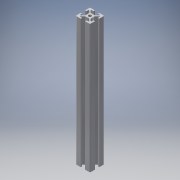
# Autodesk Inventor part: NFS5-2020-200
Saved by Autodesk Inventor 2016 (Build 200138000, 138)
## iProperties
Category: PARTsolutions
Company: MISUMI
Created: 2016-06-28
Part Number: NFS5-2020-200
Catalog Web Link: www.cadenas.de
Description: NFS5-2020, NFSB5-2020, HFS5-2020, HFSB5-2020, CAF5-2020, HFSY5-2020, NFSF5-2020, HFSF5-2020, HFSFB5-2020, NFST5-2020, HFST5-2020, HFSTB5-2020, HFSH5-2020, HFSC5-2020-HFS5 Series Aluminum Extrusions 20 Square -1 Slot-
Vendor: MISUMI
Document SubType Name: Modeling
Designer: psAdmin
Manufacturer: MISUMI
Mass: 36.2526 g
Surface Area: 351.759 cm^2
Volume: 36.2526 cm^3
Density: 2.7 g/cm^3
Material: アルミニウム 6061
Appearance: アルミニウム - フラット
PSOL_IDENT_0: {$CADENAS_DATA\23d-libs\misumi\metric\38_al_extrusions_blackets\5\hfs5_2020.prj},569 {VTYP=3D},{NB=N
PSOL_IDENT_1: FS5-2020-200},{LINA=NFS5-2020-200},{NN=NFS5-2020, NFSB5-2020, HFS5-2020, HFSB5-2020, CAF5-2020, HFSY
PSOL_IDENT_2: 5-2020, NFSF5-2020, HFSF5-2020, HFSFB5-2020, NFST5-2020, HFST5-2020, HFSTB5-2020, HFSH5-2020, HFSC5-
PSOL_IDENT_3: 2020},{DATE=31.03.2016 11:03:16},{GEOMDATE=18.03.2016 06:52:00},{VERSION=},{LINEID=10},{LINESUBID=-1
PSOL_IDENT_4: },{WBVAR=L,ALT1,ALT2,ALT4,ALT5,CP5,DL5,DR5,ALT6,ALT9,ALT10,ALT11,HP6,NHL6,DL6,NHR6,DR6,ALT7,ALT8,NH9
PSOL_IDENT_5: ,AH,BH,CH,DH,EH,NH10,AV,BV,CV,DV,EV,NH11,AP,BP,CP,DP,EP,ALT12,ALT13,Z,NH12,XA,XB,XC,XD,XE,NH13,YA,YB
PSOL_IDENT_6: ,YC,YD,YE,ALT16,HP16,DL16,DR16,ALT17,HQ17,JLP,ALT20}  {NB=NFS5-2020-200},{LINA=NFS5-2020-200},{KT=DU
PSOL_IDENT_7: MMY},{PN=NFS5-2020-200},{TPS=NFS5-2020},{MAT=6063-T5 Aluminum Alloy},{ST=Clear Anodize},{FRMW=20},{F
PSOL_IDENT_8: RMH=20},{FRD=4.2},{L=200},{MASS=0.5},{SA=183},{LX=0.742x10^4},{LY=0.742x10^4},{ALT1=},{M1=0},{DPL1=0
PSOL_IDENT_9: },{DPR1=0},{ALT1PN=},{ALT2=},{ALT2ALG= '','w/o End Tapping (Heli-Coil Insert)','LHP','with LHP (Tapp
PSOL_IDENT_10: ing on the Left (Heli-Coil Insert))','RHP','with RHP (Tapping on the Right (Heli-Coil Insert))','HPW'
PSOL_IDENT_11: ,'with HPW (Tapping on Both Ends (Heli-Coil Insert))' },{M2=0},{DP2=0},{ALT2PN=},{ALT4=},{ALT4ALG= ''
PSOL_IDENT_12: , 'w/o SC (High Precision Cut)', 'SC', 'with SC (High Precision Cut)' },{ALT4PN=},{ALT5=},{ALT5ALG= ''
PSOL_IDENT_13: ,'w/o 45 Degree Cut','1','with 45 Degree Cut' },{CP5=},{CP5ALG= '','N/A' },{DL5=},{DL5ALG= '','N/A'
PSOL_IDENT_14: },{DR5=},{DR5ALG= '','N/A' },{FRMLALT5=0},{FRMRALT5=0},{ALT5PN=},{ALT6=},{ALT6ALG= '','w/o Fastening
PSOL_IDENT_15: Location Wrench Access Hole Alterations','1','with Fastening Location Wrench Access Hole Alteration
PSOL_IDENT_16: s' },{ALT9=},{ALT9ALG= '','w/o Location Specified Wrench Access Hole Alteratons (Horizontal)','1','w
PSOL_IDENT_17: ith Location Specified Wrench Access Hole Alteratons (Horizontal)' },{ALT10=},{ALT10ALG= '','w/o Loc
PSOL_IDENT_18: ation Specified Wrench Access Hole Alteratons (Vertical)','1','with Location Specified Wrench Access
PSOL_IDENT_19: Hole Alteratons (Vertical)' },{ALT11=},{ALT11ALG= '','w/o Location Specified Wrench Access Hole Alt
PSOL_IDENT_20: eratons (Crisscross)','1','with Location Specified Wrench Access Hole Alteratons (Crisscross)' },{HP
PSOL_IDENT_21: 6=},{HP6ALG= '','N/A' },{NHL6=},{NHL6ALG= '','N/A' },{DL6=},{DL6ALG= '','N/A' },{NHR6=},{NHR6ALG= ''
PSOL_IDENT_22: ,'N/A' },{DR6=},{DR6ALG= '','N/A' },{HL6=0},{HL6D=0},{HR6=0},{HR6D=0},{J6=0},{J6D=0},{K6=0},{K6D=0},
PSOL_IDENT_23: {DD6=0.00},{DD6ALG=0},{ALT7=},{ALT7ALG= '','N/A' },{ALT8=},{ALT8ALG= '','N/A' },{ALT678PN=},{NH9=0},
PSOL_IDENT_24: {NH9MAX=5},{NH9ALG=[0]},{AH=0.0},{AHMIN=7},{AHMAX=195},{AHALG=[0]},{BH=0.0},{BHMIN=2},{BHMAX=197},{B
PSOL_IDENT_25: HALG=[0]},{CH=0.0},{CHMIN=2},{CHMAX=199},{CHALG=[0]},{DH=0.0},{DHMIN=2},{DHMAX=201},{DHALG=[0]},{EH=
PSOL_IDENT_26: 0.0},{EHMIN=2},{EHMAX=193},{EHALG=[0]},{NH10=0},{NH10MAX=5},{NH10ALG=[0]},{AV=0.0},{AVMIN=7},{AVMAX=
PSOL_IDENT_27: 195},{AVALG=[0]},{BV=0.0},{BVMIN=2},{BVMAX=197},{BVALG=[0]},{CV=0.0},{CVMIN=2},{CVMAX=199},{CVALG=[0
PSOL_IDENT_28: ]},{DV=0.0},{DVMIN=2},{DVMAX=201},{DVALG=[0]},{EV=0.0},{EVMIN=2},{EVMAX=193},{EVALG=[0]},{NH11=0},{N
PSOL_IDENT_29: H11MAX=5},{NH11ALG=[0]},{AP=0.0},{APMIN=7},{APMAX=195},{APALG=[0]},{BP=0.0},{BPMIN=2},{BPMAX=197},{B
PSOL_IDENT_30: PALG=[0]},{CP=0.0},{CPMIN=2},{CPMAX=199},{CPALG=[0]},{DP=0.0},{DPMIN=2},{DPMAX=201},{DPALG=[0]},{EP=
PSOL_IDENT_31: 0.0},{EPMIN=2},{EPMAX=193},{EPALG=[0]},{ALT9PN=},{ALT10PN=},{ALT11PN=},{ALT91011PN=},{ALT12=},{ALT12
PSOL_IDENT_32: ALG= '','w/o Counterbore Hole in Specified Position (Vertical)','1','with Counterbore Hole in Specif
PSOL_IDENT_33: ied Position (Vertical)' },{ALT13=},{ALT13ALG= '','w/o Counterbore Hole in Specified Position (Horiz
PSOL_IDENT_34: ontal)','1','with Counterbore Hole in Specified Position (Horizontal)' },{Z=},{ZALG= '','N/A' },{DD1
PSOL_IDENT_35: 2=0.0},{DD112=0.0},{NH12=0},{NH12MAX=5},{NH12ALG=[0]},{XA=0.0},{XAMIN=7},{XAMAX=195},{XAALG=[0]},{XB=
PSOL_IDENT_36: 0.0},{XBMIN=2},{XBMAX=197},{XBALG=[0]},{XC=0.0},{XCMIN=2},{XCMAX=199},{XCALG=[0]},{XD=0.0},{XDMIN=2}
PSOL_IDENT_37: ,{XDMAX=201},{XDALG=[0]},{XE=0.0},{XEMIN=2},{XEMAX=193},{XEALG=[0]},{NH13=0},{NH13MAX=5},{NH13ALG=[0
PSOL_IDENT_38: ]},{YA=0.0},{YAMIN=7},{YAMAX=195},{YAALG=[0]},{YB=0.0},{YBMIN=2},{YBMAX=197},{YBALG=[0]},{YC=0.0},{Y
PSOL_IDENT_39: CMIN=2},{YCMAX=199},{YCALG=[0]},{YD=0.0},{YDMIN=2},{YDMAX=201},{YDALG=[0]},{YE=0.0},{YEMIN=2},{YEMAX=
PSOL_IDENT_40: 193},{YEALG=[0]},{ALT12PN=},{ALT13PN=},{ALT1213PN=},{ALT16=},{ALT16ALG= '','w/o M Type Hole Alterati
PSOL_IDENT_41: on','1','with M Type Hole Alteration' },{HP16=},{HP16ALG= '','N/A' },{DL16=},{DL16ALG= '','N/A' },{D
PSOL_IDENT_42: R16=},{DR16ALG= '','N/A' },{H116=0},{D16=0.0},{ALT16PN=},{ALT17=},{ALT17ALG= '','w/o L Type Hole Alt
PSOL_IDENT_43: eration (Top)','1','with L Type Hole Alteration (Top)' },{HQ17=0},{HQ17ALG=0},{JLP=0},{JLPMIN=4.9},{
PSOL_IDENT_44: JLPMAX=0},{JLPALG=[0]},{L17=0},{D17=0.0},{ALT17PN=},{ALT20=},{ALT20PN=},{ERRORALT01=OK},{ERRORALT02=
PSOL_IDENT_45: OK},{ERRORALT05=OK},{ERRORALT06091=OK},{ERRORALT06092=OK},{ERRORALT06093=OK},{ERRORALT06094=OK},{ERR
PSOL_IDENT_46: ORALT06101=OK},{ERRORALT06102=OK},{ERRORALT06103=OK},{ERRORALT06104=OK},{ERRORALT06111=OK},{ERRORALT
PSOL_IDENT_47: 06112=OK},{ERRORALT06113=OK},{ERRORALT06114=OK},{ERRORALT06121=OK},{ERRORALT06122=OK},{ERRORALT06123=
PSOL_IDENT_48: OK},{ERRORALT06124=OK},{ERRORALT06131=OK},{ERRORALT06132=OK},{ERRORALT06133=OK},{ERRORALT06134=OK},{
PSOL_IDENT_49: ERRORALT0616=OK},{ERRORALT06171=OK},{ERRORALT06172=OK},{ERRORALT06173=OK},{ERRORALT0911=OK},{ERRORAL
PSOL_IDENT_50: T0913=OK},{ERRORALT0916=OK},{ERRORALT0917=OK},{ERRORALT1011=OK},{ERRORALT1012=OK},{ERRORALT1016=OK},
PSOL_IDENT_51: {ERRORALT1017=OK},{ERRORALT1112=OK},{ERRORALT1113=OK},{ERRORALT1116=OK},{ERRORALT1117=OK},{ERRORALT1
PSOL_IDENT_52: 216=OK},{ERRORALT1217=OK},{ERRORALT1316=OK},{ERRORALT1317=OK},{ERRORALT1617=OK},{ERRORPN=},{TFW=0}
NN: NFS5-2020, NFSB5-2020, HFS5-2020, HFSB5-2020, CAF5-2020, HFSY5-2020, NFSF5-2020, HFSF5-2020, HFSFB5-2020, NFST5-2020, HFST5-2020, HFSTB5-2020, HFSH5-2020, HFSC5-2020
NT: HFS5 Series Aluminum Extrusions 20 Square -1 Slot-
NB: NFS5-2020-200
NBSYN: $PN.
LINA: NFS5-2020-200
PN: NFS5-2020-200
TPS: NFS5-2020
MAT: 6063-T5 Aluminum Alloy
ST: Clear Anodize
L: 200
MASS: 0.5
SA: 183
LX: 0.742x10^4
LY: 0.742x10^4
ALT1: w/o End Tapping
M1: 0
DPL1: 0
DPR1: 0
ALT2: w/o End Tapping (Heli-Coil Insert)
M2: 0
DP2: 0
ALT4: w/o SC (High Precision Cut)
ALT5: w/o 45 Degree Cut
CP5: N/A
DL5: N/A
DR5: N/A
ALT6: w/o Fastening Location Wrench Access Hole Alterations
ALT9: w/o Location Specified Wrench Access Hole Alteratons (Horizontal)
ALT10: w/o Location Specified Wrench Access Hole Alteratons (Vertical)
ALT11: w/o Location Specified Wrench Access Hole Alteratons (Crisscross)
HP6: N/A
NHL6: N/A
DL6: N/A
NHR6: N/A
DR6: N/A
HL6D: 0
HR6D: 0
J6D: 0
K6D: 0
DD6: 0.00
ALT7: N/A
ALT8: N/A
NH9: 0
AH: 0.0
BH: 0.0
CH: 0.0
DH: 0.0
EH: 0.0
NH10: 0
AV: 0.0
BV: 0.0
CV: 0.0
DV: 0.0
EV: 0.0
NH11: 0
AP: 0.0
BP: 0.0
CP: 0.0
DP: 0.0
EP: 0.0
ALT12: w/o Counterbore Hole in Specified Position (Vertical)
ALT13: w/o Counterbore Hole in Specified Position (Horizontal)
Z: N/A
DD12: 0.0
DD112: 0.0
NH12: 0
XA: 0.0
XB: 0.0
XC: 0.0
XD: 0.0
XE: 0.0
NH13: 0
YA: 0.0
YB: 0.0
YC: 0.0
YD: 0.0
YE: 0.0
ALT16: w/o M Type Hole Alteration
HP16: N/A
DL16: N/A
DR16: N/A
H116: 0
D16: 0.0
ALT17: w/o L Type Hole Alteration (Top)
HQ17: 0
JLP: 0
D17: 0.0
ALT20: w/o CW (End Face C Chamfering)
SUPPLIER: MISUMI
ARTICLENO: NFS5-2020-200
BOMINFO: NFS5-2020-200
CREATOR: CADENAS GmbH
Title: NFS5-2020-200
Author: Cadenas PARTsolutions
Comments: HFS5 Series Aluminum Extrusions 20 Square -1 Slot-
Autodesk Inventor part; units mm, degrees
ref_plane "YZ Plane" through (0, 0, 0) normal (1, 0, 0) x (0, 1, 0)
ref_plane "XZ Plane" through (0, 0, 0) normal (0, 1, 0) x (-1, 0, 0)
ref_plane "XY Plane" through (0, 0, 0) normal (0, 0, 1) x (1, 0, 0)
sketch "Sketch_75" plane through (0, 0, 0) normal (0, 0, 1) x (1, 0, 0)
  line L0 (-10, 3) -> (-8, 3)
  line L1 (-8, 3) -> (-8, 6)
  line L2 (-8, 6) -> (-7.0607, 6)
  line L3 (-7.0607, 6) -> (-4, 2.9393)
  line L4 (-4, 2.9393) -> (-4, 0.6536)
  arc A0 (-4, 0.6536) -> (-3.933, 0.4036) centre (-3.5, 0.6536) ccw
  line L5 (-3.933, 0.4036) -> (-3.7, 0)
  line L6 (-3.7, 0) -> (-3.933, -0.4036)
  arc A1 (-3.933, -0.4036) -> (-3.933, -0.9036) centre (-3.5, -0.6536) ccw
  line L7 (-3.933, -0.9036) -> (-3.751, -1.2189)
  line L8 (-3.751, -1.2189) -> (-4, -2.5)
  line L9 (-4, -2.5) -> (-4, -2.9393)
  line L10 (-4, -2.9393) -> (-7.0607, -6)
  line L11 (-7.0607, -6) -> (-8, -6)
  line L12 (-8, -6) -> (-8, -3)
  line L13 (-8, -3) -> (-10, -3)
  line L14 (-10, -3) -> (-10, -9)
  arc A2 (-10, -9) -> (-9, -10) centre (-9, -9) ccw
  line L15 (-9, -10) -> (-3, -10)
  line L16 (-3, -10) -> (-3, -8)
  line L17 (-3, -8) -> (-6, -8)
  line L18 (-6, -8) -> (-6, -7.0607)
  line L19 (-6, -7.0607) -> (-2.9393, -4)
  line L20 (-2.9393, -4) -> (-0.6536, -4)
  arc A3 (-0.6536, -4) -> (-0.4036, -3.933) centre (-0.6536, -3.5) ccw
  line L21 (-0.4036, -3.933) -> (0, -3.7)
  line L22 (0, -3.7) -> (0.4036, -3.933)
  arc A4 (0.4036, -3.933) -> (0.9036, -3.933) centre (0.6536, -3.5) ccw
  line L23 (0.9036, -3.933) -> (1.2189, -3.751)
  line L24 (1.2189, -3.751) -> (2.5, -4)
  line L25 (2.5, -4) -> (2.9393, -4)
  line L26 (2.9393, -4) -> (6, -7.0607)
  line L27 (6, -7.0607) -> (6, -8)
  line L28 (6, -8) -> (3, -8)
  line L29 (3, -8) -> (3, -10)
  line L30 (3, -10) -> (9, -10)
  arc A5 (9, -10) -> (10, -9) centre (9, -9) ccw
  line L31 (10, -9) -> (10, -3)
  line L32 (10, -3) -> (8, -3)
  line L33 (8, -3) -> (8, -6)
  line L34 (8, -6) -> (7.0607, -6)
  line L35 (7.0607, -6) -> (4, -2.9393)
  line L36 (4, -2.9393) -> (4, -0.6536)
  arc A6 (4, -0.6536) -> (3.933, -0.4036) centre (3.5, -0.6536) ccw
  line L37 (3.933, -0.4036) -> (3.7, 0)
  line L38 (3.7, 0) -> (3.933, 0.4036)
  arc A7 (3.933, 0.4036) -> (3.933, 0.9036) centre (3.5, 0.6536) ccw
  line L39 (3.933, 0.9036) -> (3.751, 1.2189)
  line L40 (3.751, 1.2189) -> (4, 2.5)
  line L41 (4, 2.5) -> (4, 2.9393)
  line L42 (4, 2.9393) -> (7.0607, 6)
  line L43 (7.0607, 6) -> (8, 6)
  line L44 (8, 6) -> (8, 3)
  line L45 (8, 3) -> (10, 3)
  line L46 (10, 3) -> (10, 9)
  arc A8 (10, 9) -> (9, 10) centre (9, 9) ccw
  line L47 (9, 10) -> (3, 10)
  line L48 (3, 10) -> (3, 8)
  line L49 (3, 8) -> (6, 8)
  line L50 (6, 8) -> (6, 7.0607)
  line L51 (6, 7.0607) -> (2.9393, 4)
  line L52 (2.9393, 4) -> (0.6536, 4)
  arc A9 (0.6536, 4) -> (0.4036, 3.933) centre (0.6536, 3.5) ccw
  line L53 (0.4036, 3.933) -> (0, 3.7)
  line L54 (0, 3.7) -> (-0.4036, 3.933)
  arc A10 (-0.4036, 3.933) -> (-0.9036, 3.933) centre (-0.6536, 3.5) ccw
  line L55 (-0.9036, 3.933) -> (-1.2189, 3.751)
  line L56 (-1.2189, 3.751) -> (-2.5, 4)
  line L57 (-2.5, 4) -> (-2.9393, 4)
  line L58 (-2.9393, 4) -> (-6, 7.0607)
  line L59 (-6, 7.0607) -> (-6, 8)
  line L60 (-6, 8) -> (-3, 8)
  line L61 (-3, 8) -> (-3, 10)
  line L62 (-3, 10) -> (-9, 10)
  arc A11 (-9, 10) -> (-10, 9) centre (-9, 9) ccw
  line L63 (-10, 9) -> (-10, 3)
  constraints: 128 end point, 24 point on circle, 12 centre point
extrude "Extrusion1" add sketch "Sketch_75" against normal blind 180
sketch "Sketch2" plane through (0, 0, -180) normal (0, 0, -1) x (-1, 0, 0)
  point P0 (0, 0)
hole "Hole1" at (0, 0, -180) direction (0, 0, 1) diameter 4.2 depth 200
ref_plane "C1_XY" through (0, 0, 0) normal (0, 0, 1) x (1, 0, 0)
ref_plane "C1_YZ" through (0, 0, 0) normal (1, 0, 0) x (0, 1, 0)
ref_plane "C1_ZX" through (0, 0, 0) normal (0, 1, 0) x (0, 0, 1)
body "Solid1"
